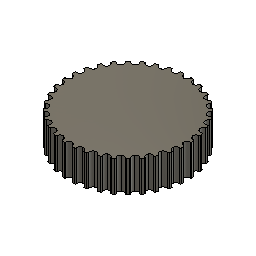
ES Gear v2 (Autodesk Fusion 360 design; units mm, degrees)
Autodesk Fusion 360 part; units mm, degrees
sketch "Sketch1" plane through (0, 0, 0) normal (0, 1, 0) x (1, 0, 0)
  circle A0 centre (0, 0) radius 39.215 construction
  circle A1 centre (0, 0) radius 37.155 construction
  line L0 (0, 0) -> (0, 45) construction
  line L1 (0, 0) -> (5.7267, 45.3317) construction
  line L2 (0, 0) -> (45.692, 0) construction
  circle A2 centre (0, 38.68) radius 1.525 construction
  circle A3 centre (4.8479, 38.375) radius 1.525 construction
  circle A4 centre (1.9542, 38.7357) radius 0.43 construction
  circle A5 centre (2.9161, 38.6752) radius 0.43 construction
  arc A6 (3.341, 38.6092) -> (4.6568, 36.862) centre (4.8479, 38.375) ccw
  arc A7 (3.341, 38.6092) -> (2.9484, 39.104) centre (2.9161, 38.6752) ccw
  arc A8 (1.9759, 39.1652) -> (1.5244, 38.7235) centre (1.9542, 38.7357) ccw
  arc A9 (0, 37.155) -> (1.5244, 38.7235) centre (0, 38.68) ccw
  line L3 (1.9759, 39.1652) -> (2.9484, 39.104)
  circle A10 centre (0, 0) radius 26.7515 construction
  circle A11 centre (0, 0) radius 28.711 construction
  arc A12 (1.9759, 39.1652) -> (1.5244, 38.7235) centre (1.9542, 38.7357) ccw
  line L4 (1.9759, 39.1652) -> (2.9484, 39.104)
  arc A13 (3.341, 38.6092) -> (2.9484, 39.104) centre (2.9161, 38.6752) ccw
  arc A14 (3.341, 38.6092) -> (4.6568, 36.862) centre (4.8479, 38.375) ccw
  arc A15 (0, 37.155) -> (1.5244, 38.7235) centre (0, 38.68) ccw
  arc A16 (0, 26.752) -> (1.5622, 28.2828) centre (0.0373, 28.2765) ccw
  arc A17 (2.0244, 28.7133) -> (1.5622, 28.2828) centre (1.9922, 28.2845) ccw
  line L5 (2.0244, 28.7133) -> (2.9951, 28.6284)
  arc A18 (3.3755, 28.1241) -> (2.9951, 28.6284) centre (2.9524, 28.2005) ccw
  arc A19 (3.3755, 28.1241) -> (4.6454, 26.3456) centre (4.8762, 27.853) ccw
  arc A20 (-4.6454, 26.3456) -> (-3.3727, 28.1244) centre (-4.8735, 27.8534) ccw
  arc A21 (-2.9924, 28.6286) -> (-3.3727, 28.1244) centre (-2.9496, 28.2008) ccw
  line L6 (-2.9924, 28.6286) -> (-2.0216, 28.7136)
  arc A22 (-1.5595, 28.283) -> (-2.0216, 28.7136) centre (-1.9895, 28.2848) ccw
  arc A23 (-1.5595, 28.283) -> (0, 26.752) centre (-0.0345, 28.2766) ccw
  arc A24 (-9.1497, 25.1387) -> (-8.2052, 27.1114) centre (-9.6361, 26.584) ccw
  arc A25 (-7.9182, 27.6741) -> (-8.2052, 27.1114) centre (-7.8018, 27.2601) ccw
  line L7 (-7.9182, 27.6741) -> (-6.977, 27.9263)
  arc A26 (-6.4471, 27.5825) -> (-6.977, 27.9263) centre (-6.8708, 27.5096) ccw
  arc A27 (-6.4471, 27.5825) -> (-4.6454, 26.3456) centre (-4.9441, 27.841) ccw
  arc A28 (-13.376, 23.1679) -> (-12.7884, 25.2747) centre (-14.106, 24.5068) ccw
  arc A29 (-12.6035, 25.8787) -> (-12.7884, 25.2747) centre (-12.4169, 25.4912) ccw
  line L8 (-12.6035, 25.8787) -> (-11.7203, 26.2905)
  arc A30 (-11.1388, 26.044) -> (-11.7203, 26.2905) centre (-11.5434, 25.8985) ccw
  arc A31 (-11.1388, 26.044) -> (-9.1497, 25.1387) centre (-9.7036, 26.5595) ccw
  arc A32 (-17.1959, 20.4932) -> (-16.9831, 22.67) centre (-18.1473, 21.685) ccw
  arc A33 (-16.9058, 23.2969) -> (-16.9831, 22.67) centre (-16.6548, 22.9478) ccw
  line L9 (-16.9058, 23.2969) -> (-16.1076, 23.8559)
  arc A34 (-15.492, 23.7141) -> (-16.1076, 23.8559) centre (-15.8653, 23.5006) ccw
  arc A35 (-15.492, 23.7141) -> (-13.376, 23.1679) centre (-14.1682, 24.471) ccw
  arc A36 (-20.4932, 17.1959) -> (-20.6617, 19.3766) centre (-21.6371, 18.2044) ccw
  arc A37 (-20.6944, 20.0073) -> (-20.6617, 19.3766) centre (-20.3866, 19.7071) ccw
  line L10 (-20.6944, 20.0073) -> (-20.0054, 20.6964)
  arc A38 (-19.3746, 20.6636) -> (-20.0054, 20.6964) centre (-19.7051, 20.3886) ccw
  arc A39 (-19.3746, 20.6636) -> (-17.1959, 20.4932) centre (-18.2023, 21.639) ccw
  arc A40 (-23.1679, 13.376) -> (-23.7125, 15.4943) centre (-24.4696, 14.1705) ccw
  arc A41 (-23.8543, 16.1098) -> (-23.7125, 15.4943) centre (-23.499, 15.8676) ccw
  line L11 (-23.8543, 16.1098) -> (-23.2953, 16.9081)
  arc A42 (-22.6685, 16.9853) -> (-23.2953, 16.9081) centre (-22.9462, 16.6571) ccw
  arc A43 (-22.6685, 16.9853) -> (-20.4932, 17.1959) centre (-21.6833, 18.1494) ccw
  arc A44 (-25.1387, 9.1497) -> (-26.0428, 11.1413) centre (-26.5585, 9.7062) ccw
  arc A45 (-26.2893, 11.7228) -> (-26.0428, 11.1413) centre (-25.8974, 11.546) ccw
  line L12 (-26.2893, 11.7228) -> (-25.8775, 12.606)
  arc A46 (-25.2735, 12.791) -> (-25.8775, 12.606) centre (-25.4901, 12.4194) ccw
  arc A47 (-25.2735, 12.791) -> (-23.1679, 13.376) centre (-24.5055, 14.1084) ccw
  arc A48 (-26.3456, 4.6454) -> (-27.5818, 6.4498) centre (-27.8405, 4.9469) ccw
  arc A49 (-27.9256, 6.9797) -> (-27.5818, 6.4498) centre (-27.5089, 6.8735) ccw
  line L13 (-27.9256, 6.9797) -> (-27.6734, 7.9209)
  arc A50 (-27.1107, 8.2079) -> (-27.6734, 7.9209) centre (-27.2594, 7.8045) ccw
  arc A51 (-27.1107, 8.2079) -> (-25.1387, 9.1497) centre (-26.5831, 9.6388) ccw
  arc A52 (-26.752, 0) -> (-28.2828, 1.5622) centre (-28.2765, 0.0373) ccw
  arc A53 (-28.7133, 2.0244) -> (-28.2828, 1.5622) centre (-28.2845, 1.9922) ccw
  line L14 (-28.7133, 2.0244) -> (-28.6284, 2.9951)
  arc A54 (-28.1241, 3.3755) -> (-28.6284, 2.9951) centre (-28.2005, 2.9524) ccw
  arc A55 (-28.1241, 3.3755) -> (-26.3456, 4.6454) centre (-27.853, 4.8762) ccw
  arc A56 (-26.3456, -4.6454) -> (-28.1244, -3.3727) centre (-27.8534, -4.8735) ccw
  arc A57 (-28.6286, -2.9924) -> (-28.1244, -3.3727) centre (-28.2008, -2.9496) ccw
  line L15 (-28.6286, -2.9924) -> (-28.7136, -2.0216)
  arc A58 (-28.283, -1.5595) -> (-28.7136, -2.0216) centre (-28.2848, -1.9895) ccw
  arc A59 (-28.283, -1.5595) -> (-26.752, 0) centre (-28.2766, -0.0345) ccw
  arc A60 (-25.1387, -9.1497) -> (-27.1114, -8.2052) centre (-26.584, -9.6361) ccw
  arc A61 (-27.6741, -7.9182) -> (-27.1114, -8.2052) centre (-27.2601, -7.8018) ccw
  line L16 (-27.6741, -7.9182) -> (-27.9263, -6.977)
  arc A62 (-27.5825, -6.4471) -> (-27.9263, -6.977) centre (-27.5096, -6.8708) ccw
  arc A63 (-27.5825, -6.4471) -> (-26.3456, -4.6454) centre (-27.841, -4.9441) ccw
  arc A64 (-23.1679, -13.376) -> (-25.2747, -12.7884) centre (-24.5068, -14.106) ccw
  arc A65 (-25.8787, -12.6035) -> (-25.2747, -12.7884) centre (-25.4912, -12.4169) ccw
  line L17 (-25.8787, -12.6035) -> (-26.2905, -11.7203)
  arc A66 (-26.044, -11.1388) -> (-26.2905, -11.7203) centre (-25.8985, -11.5434) ccw
  arc A67 (-26.044, -11.1388) -> (-25.1387, -9.1497) centre (-26.5595, -9.7036) ccw
  arc A68 (-20.4932, -17.1959) -> (-22.67, -16.9831) centre (-21.685, -18.1473) ccw
  arc A69 (-23.2969, -16.9058) -> (-22.67, -16.9831) centre (-22.9478, -16.6548) ccw
  line L18 (-23.2969, -16.9058) -> (-23.8559, -16.1076)
  arc A70 (-23.7141, -15.492) -> (-23.8559, -16.1076) centre (-23.5006, -15.8653) ccw
  arc A71 (-23.7141, -15.492) -> (-23.1679, -13.376) centre (-24.471, -14.1682) ccw
  arc A72 (-17.1959, -20.4932) -> (-19.3766, -20.6617) centre (-18.2044, -21.6371) ccw
  arc A73 (-20.0073, -20.6944) -> (-19.3766, -20.6617) centre (-19.7071, -20.3866) ccw
  line L19 (-20.0073, -20.6944) -> (-20.6964, -20.0054)
  arc A74 (-20.6636, -19.3746) -> (-20.6964, -20.0054) centre (-20.3886, -19.7051) ccw
  arc A75 (-20.6636, -19.3746) -> (-20.4932, -17.1959) centre (-21.639, -18.2023) ccw
  arc A76 (-13.376, -23.1679) -> (-15.4943, -23.7125) centre (-14.1705, -24.4696) ccw
  arc A77 (-16.1098, -23.8543) -> (-15.4943, -23.7125) centre (-15.8676, -23.499) ccw
  line L20 (-16.1098, -23.8543) -> (-16.9081, -23.2953)
  arc A78 (-16.9853, -22.6685) -> (-16.9081, -23.2953) centre (-16.6571, -22.9462) ccw
  arc A79 (-16.9853, -22.6685) -> (-17.1959, -20.4932) centre (-18.1494, -21.6833) ccw
  arc A80 (-9.1497, -25.1387) -> (-11.1413, -26.0428) centre (-9.7062, -26.5585) ccw
  arc A81 (-11.7228, -26.2893) -> (-11.1413, -26.0428) centre (-11.546, -25.8974) ccw
  line L21 (-11.7228, -26.2893) -> (-12.606, -25.8775)
  arc A82 (-12.791, -25.2735) -> (-12.606, -25.8775) centre (-12.4194, -25.4901) ccw
  arc A83 (-12.791, -25.2735) -> (-13.376, -23.1679) centre (-14.1084, -24.5055) ccw
  arc A84 (-4.6454, -26.3456) -> (-6.4498, -27.5818) centre (-4.9469, -27.8405) ccw
  arc A85 (-6.9797, -27.9256) -> (-6.4498, -27.5818) centre (-6.8735, -27.5089) ccw
  line L22 (-6.9797, -27.9256) -> (-7.9209, -27.6734)
  arc A86 (-8.2079, -27.1107) -> (-7.9209, -27.6734) centre (-7.8045, -27.2594) ccw
  arc A87 (-8.2079, -27.1107) -> (-9.1497, -25.1387) centre (-9.6388, -26.5831) ccw
  arc A88 (0, -26.752) -> (-1.5622, -28.2828) centre (-0.0373, -28.2765) ccw
  arc A89 (-2.0244, -28.7133) -> (-1.5622, -28.2828) centre (-1.9922, -28.2845) ccw
  line L23 (-2.0244, -28.7133) -> (-2.9951, -28.6284)
  arc A90 (-3.3755, -28.1241) -> (-2.9951, -28.6284) centre (-2.9524, -28.2005) ccw
  arc A91 (-3.3755, -28.1241) -> (-4.6454, -26.3456) centre (-4.8762, -27.853) ccw
  arc A92 (4.6454, -26.3456) -> (3.3727, -28.1244) centre (4.8735, -27.8534) ccw
  arc A93 (2.9924, -28.6286) -> (3.3727, -28.1244) centre (2.9496, -28.2008) ccw
  line L24 (2.9924, -28.6286) -> (2.0216, -28.7136)
  arc A94 (1.5595, -28.283) -> (2.0216, -28.7136) centre (1.9895, -28.2848) ccw
  arc A95 (1.5595, -28.283) -> (0, -26.752) centre (0.0345, -28.2766) ccw
  arc A96 (9.1497, -25.1387) -> (8.2052, -27.1114) centre (9.6361, -26.584) ccw
  arc A97 (7.9182, -27.6741) -> (8.2052, -27.1114) centre (7.8018, -27.2601) ccw
  line L25 (7.9182, -27.6741) -> (6.977, -27.9263)
  arc A98 (6.4471, -27.5825) -> (6.977, -27.9263) centre (6.8708, -27.5096) ccw
  arc A99 (6.4471, -27.5825) -> (4.6454, -26.3456) centre (4.9441, -27.841) ccw
  arc A100 (13.376, -23.1679) -> (12.7884, -25.2747) centre (14.106, -24.5068) ccw
  arc A101 (12.6035, -25.8787) -> (12.7884, -25.2747) centre (12.4169, -25.4912) ccw
  line L26 (12.6035, -25.8787) -> (11.7203, -26.2905)
  arc A102 (11.1388, -26.044) -> (11.7203, -26.2905) centre (11.5434, -25.8985) ccw
  arc A103 (11.1388, -26.044) -> (9.1497, -25.1387) centre (9.7036, -26.5595) ccw
  arc A104 (17.1959, -20.4932) -> (16.9831, -22.67) centre (18.1473, -21.685) ccw
  arc A105 (16.9058, -23.2969) -> (16.9831, -22.67) centre (16.6548, -22.9478) ccw
  line L27 (16.9058, -23.2969) -> (16.1076, -23.8559)
  arc A106 (15.492, -23.7141) -> (16.1076, -23.8559) centre (15.8653, -23.5006) ccw
  arc A107 (15.492, -23.7141) -> (13.376, -23.1679) centre (14.1682, -24.471) ccw
  arc A108 (20.4932, -17.1959) -> (20.6617, -19.3766) centre (21.6371, -18.2044) ccw
  arc A109 (20.6944, -20.0073) -> (20.6617, -19.3766) centre (20.3866, -19.7071) ccw
  line L28 (20.6944, -20.0073) -> (20.0054, -20.6964)
  arc A110 (19.3746, -20.6636) -> (20.0054, -20.6964) centre (19.7051, -20.3886) ccw
  arc A111 (19.3746, -20.6636) -> (17.1959, -20.4932) centre (18.2023, -21.639) ccw
  arc A112 (23.1679, -13.376) -> (23.7125, -15.4943) centre (24.4696, -14.1705) ccw
  arc A113 (23.8543, -16.1098) -> (23.7125, -15.4943) centre (23.499, -15.8676) ccw
  line L29 (23.8543, -16.1098) -> (23.2953, -16.9081)
  arc A114 (22.6685, -16.9853) -> (23.2953, -16.9081) centre (22.9462, -16.6571) ccw
  arc A115 (22.6685, -16.9853) -> (20.4932, -17.1959) centre (21.6833, -18.1494) ccw
  arc A116 (25.1387, -9.1497) -> (26.0428, -11.1413) centre (26.5585, -9.7062) ccw
  arc A117 (26.2893, -11.7228) -> (26.0428, -11.1413) centre (25.8974, -11.546) ccw
  line L30 (26.2893, -11.7228) -> (25.8775, -12.606)
  arc A118 (25.2735, -12.791) -> (25.8775, -12.606) centre (25.4901, -12.4194) ccw
  arc A119 (25.2735, -12.791) -> (23.1679, -13.376) centre (24.5055, -14.1084) ccw
  arc A120 (26.3456, -4.6454) -> (27.5818, -6.4498) centre (27.8405, -4.9469) ccw
  arc A121 (27.9256, -6.9797) -> (27.5818, -6.4498) centre (27.5089, -6.8735) ccw
  line L31 (27.9256, -6.9797) -> (27.6734, -7.9209)
  arc A122 (27.1107, -8.2079) -> (27.6734, -7.9209) centre (27.2594, -7.8045) ccw
  arc A123 (27.1107, -8.2079) -> (25.1387, -9.1497) centre (26.5831, -9.6388) ccw
  arc A124 (26.752, 0) -> (28.2828, -1.5622) centre (28.2765, -0.0373) ccw
  arc A125 (28.7133, -2.0244) -> (28.2828, -1.5622) centre (28.2845, -1.9922) ccw
  line L32 (28.7133, -2.0244) -> (28.6284, -2.9951)
  arc A126 (28.1241, -3.3755) -> (28.6284, -2.9951) centre (28.2005, -2.9524) ccw
  arc A127 (28.1241, -3.3755) -> (26.3456, -4.6454) centre (27.853, -4.8762) ccw
  arc A128 (26.3456, 4.6454) -> (28.1244, 3.3727) centre (27.8534, 4.8735) ccw
  arc A129 (28.6286, 2.9924) -> (28.1244, 3.3727) centre (28.2008, 2.9496) ccw
  line L33 (28.6286, 2.9924) -> (28.7136, 2.0216)
  arc A130 (28.283, 1.5595) -> (28.7136, 2.0216) centre (28.2848, 1.9895) ccw
  arc A131 (28.283, 1.5595) -> (26.752, 0) centre (28.2766, 0.0345) ccw
  arc A132 (25.1387, 9.1497) -> (27.1114, 8.2052) centre (26.584, 9.6361) ccw
  arc A133 (27.6741, 7.9182) -> (27.1114, 8.2052) centre (27.2601, 7.8018) ccw
  line L34 (27.6741, 7.9182) -> (27.9263, 6.977)
  arc A134 (27.5825, 6.4471) -> (27.9263, 6.977) centre (27.5096, 6.8708) ccw
  arc A135 (27.5825, 6.4471) -> (26.3456, 4.6454) centre (27.841, 4.9441) ccw
  arc A136 (23.1679, 13.376) -> (25.2747, 12.7884) centre (24.5068, 14.106) ccw
  arc A137 (25.8787, 12.6035) -> (25.2747, 12.7884) centre (25.4912, 12.4169) ccw
  line L35 (25.8787, 12.6035) -> (26.2905, 11.7203)
  arc A138 (26.044, 11.1388) -> (26.2905, 11.7203) centre (25.8985, 11.5434) ccw
  arc A139 (26.044, 11.1388) -> (25.1387, 9.1497) centre (26.5595, 9.7036) ccw
  arc A140 (20.4932, 17.1959) -> (22.67, 16.9831) centre (21.685, 18.1473) ccw
  arc A141 (23.2969, 16.9058) -> (22.67, 16.9831) centre (22.9478, 16.6548) ccw
  line L36 (23.2969, 16.9058) -> (23.8559, 16.1076)
  arc A142 (23.7141, 15.492) -> (23.8559, 16.1076) centre (23.5006, 15.8653) ccw
  arc A143 (23.7141, 15.492) -> (23.1679, 13.376) centre (24.471, 14.1682) ccw
  arc A144 (17.1959, 20.4932) -> (19.3766, 20.6617) centre (18.2044, 21.6371) ccw
  arc A145 (20.0073, 20.6944) -> (19.3766, 20.6617) centre (19.7071, 20.3866) ccw
  line L37 (20.0073, 20.6944) -> (20.6964, 20.0054)
  arc A146 (20.6636, 19.3746) -> (20.6964, 20.0054) centre (20.3886, 19.7051) ccw
  arc A147 (20.6636, 19.3746) -> (20.4932, 17.1959) centre (21.639, 18.2023) ccw
  arc A148 (13.376, 23.1679) -> (15.4943, 23.7125) centre (14.1705, 24.4696) ccw
  arc A149 (16.1098, 23.8543) -> (15.4943, 23.7125) centre (15.8676, 23.499) ccw
  line L38 (16.1098, 23.8543) -> (16.9081, 23.2953)
  arc A150 (16.9853, 22.6685) -> (16.9081, 23.2953) centre (16.6571, 22.9462) ccw
  arc A151 (16.9853, 22.6685) -> (17.1959, 20.4932) centre (18.1494, 21.6833) ccw
  arc A152 (9.1497, 25.1387) -> (11.1413, 26.0428) centre (9.7062, 26.5585) ccw
  arc A153 (11.7228, 26.2893) -> (11.1413, 26.0428) centre (11.546, 25.8974) ccw
  line L39 (11.7228, 26.2893) -> (12.606, 25.8775)
  arc A154 (12.791, 25.2735) -> (12.606, 25.8775) centre (12.4194, 25.4901) ccw
  arc A155 (12.791, 25.2735) -> (13.376, 23.1679) centre (14.1084, 24.5055) ccw
  arc A156 (4.6454, 26.3456) -> (6.4498, 27.5818) centre (4.9469, 27.8405) ccw
  arc A157 (6.9797, 27.9256) -> (6.4498, 27.5818) centre (6.8735, 27.5089) ccw
  line L40 (6.9797, 27.9256) -> (7.9209, 27.6734)
  arc A158 (8.2079, 27.1107) -> (7.9209, 27.6734) centre (7.8045, 27.2594) ccw
  arc A159 (8.2079, 27.1107) -> (9.1497, 25.1387) centre (9.6388, 26.5831) ccw
  dimension "d1" = 78.43
  dimension "d2" = 74.31
  dimension "d3" = 82.8
  dimension "d4" = 3.05
  dimension "d5" = 3.05
  dimension "d6" = 0.86
  dimension "d7" = 0.86
  dimension "d8" = 53.503
  dimension "d9" = 57.422
  dimension "d11" = 360
  constraint coincident A0.centre A1.centre
  constraint concentric A0 A1
  constraint vertical L0
  constraint horizontal L2
  constraint tangent A2 A4
  constraint tangent A0 A4
  constraint tangent A3 A5
  constraint tangent A0 A5
  constraint coincident A5 A6.start
  constraint coincident A3 A6.end
  constraint coincident A1 A6.end
  constraint coincident L1 A6.end
  constraint coincident A3.centre A6.centre
  constraint coincident A0 A7.end
  constraint coincident A5.centre A7.centre
  constraint coincident A2 A8.end
  constraint coincident A4 A8.end
  constraint coincident A0 A8.start
  constraint coincident A4 A8.start
  constraint coincident A4.centre A8.centre
  constraint coincident A1 A9.start
  constraint coincident L0 A9.start
  measures "d1" diameter of A0
  measures "d2" diameter of A1
  measures "d3" angle of L1 L2
  measures "d4" diameter of A2
  measures "d5" diameter of A3
  measures "d6" diameter of A4
  measures "d7" diameter of A5
  measures "d8" diameter of A10
  measures "d9" diameter of A11
extrude "Extrude1" add sketch "Sketch1" along normal blind 15
equation "d3 = 90 deg - 7.2 deg"
equation "d9 = 53.302 mm + 4.12 mm"
